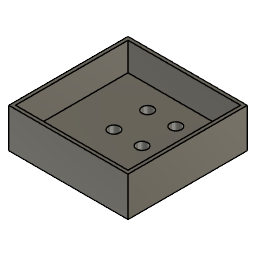
MORSE2 (Autodesk Fusion 360 design; units mm, degrees)
part number: 2026-03-12-14-39-51-275
Autodesk Fusion 360 part; units mm, degrees
sketch "Sketch1" plane through (0, 0, 0) normal (0, 0, 1) x (1, 0, 0)
  line L0 (-50, 50) -> (50, 50)
  line L1 (50, 50) -> (50, -50)
  line L2 (50, -50) -> (-50, -50)
  line L3 (-50, -50) -> (-50, 50)
  line L4 (-50, 50) -> (50, -50) construction
  line L5 (50, 50) -> (-50, -50) construction
  line L6 (53, 53) -> (53, -53)
  line L7 (53, -53) -> (-53, -53)
  line L8 (-53, -53) -> (-53, 53)
  line L9 (-53, 53) -> (53, 53)
  dimension "d1" = -3
  constraint horizontal L0
  constraint perpendicular L0 L1
  constraint parallel L0 L2
  constraint parallel L1 L3
  constraint coincident L4 origin
  constraint coincident L5 origin
extrude "Extrude1" add sketch "Sketch1" along normal blind 35
extrude "Extrude2" add sketch "Sketch1" along normal blind 10 contours L0 L1 L2 L3
sketch "Sketch3" plane through (0, 0, 0) normal (0, 0, -1) x (1, 0, 0)
  line L0 (-53, 53) -> (-53, -53)
  line L1 (-53, -53) -> (53, -53)
  line L2 (53, -53) -> (53, 53)
  line L3 (53, 53) -> (-53, 53)
  circle A0 centre (-12.5, 0) radius 5
  circle A1 centre (12.5, 0) radius 5
  circle A2 centre (-12.5, 30) radius 5
  circle A3 centre (12.5, 30) radius 5
  circle A4 centre (-12.5, -30) radius 5
  circle A5 centre (12.5, -30) radius 5
  dimension "d6" = 10
  dimension "d7" = 10
  dimension "d8" = 25
  dimension "d9" = 12.5
  dimension "d12" = 0
  dimension "d13" = 30
  dimension "d16" = 0
  dimension "d17" = -30
  constraint horizontal A0.centre A1.centre
  constraint horizontal origin A0.centre
  measures "d6" diameter of A0
  measures "d7" diameter of A1
  measures "d8" distance of A0.centre A1.centre
  measures "d9" horizontal distance of origin A1.centre
extrude "Extrude3" cut sketch "Sketch3" against normal blind 10 contours A0 | A1 | A2 | A3 | A4 | A5
